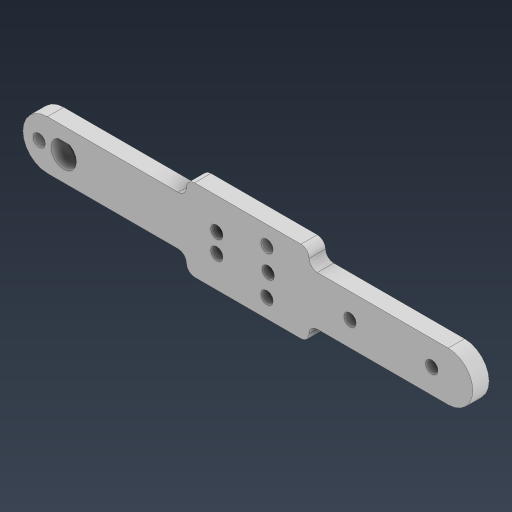
# Autodesk Inventor part: Arm1_3D
Saved by Autodesk Inventor 2023 (Build 270158000, 158)
## iProperties
Created: 2024-02-10
Part Number: Arm1_3D
Material: Generic
Document SubType Name: Modeling
Designer: victo
Density: 1 g/cm^3
Appearance: Default
Author: victo
Autodesk Inventor part; units mm, degrees
ref_plane "YZ Plane" through (0, 0, 0) normal (1, 0, 0) x (0, 1, 0)
ref_plane "XZ Plane" through (0, 0, 0) normal (0, 1, 0) x (-1, 0, 0)
ref_plane "XY Plane" through (0, 0, 0) normal (0, 0, 1) x (1, 0, 0)
sketch "Sketch1" plane through (0, 0, 0) normal (0, 0, 1) x (1, 0, 0)
  line L0 (0, 0) -> (90, 0) construction
  line L1 (0, -10) -> (90, -10)
  line L2 (90, 10) -> (0, 10)
  arc A0 (0, 10) -> (0, -10) centre (0, 0) ccw
  arc A1 (90, -10) -> (90, 10) centre (90, 0) ccw
  line L3 (0, 0) -> (90, 0) construction
  circle A2 centre (0, 0) radius 3.1
  circle A3 centre (-6, 0) radius 1.5
  circle A4 centre (0, 0) radius 37.5 construction
  circle A5 centre (0, 0) radius 50 construction
  circle A6 centre (37.4301, 2.2893) radius 1.5
  circle A7 centre (37.4301, -2.2893) radius 1.5
  circle A8 centre (50, 0) radius 1.5
  circle A9 centre (49.7028, 5.4433) radius 1.5
  circle A10 centre (49.7028, -5.4433) radius 1.5
  line L4 (37.4301, 2.2893) -> (0, 0) construction
  line L5 (0, 0) -> (49.7028, 5.4433) construction
  line L6 (37.4301, -2.2893) -> (0, 0) construction
  line L7 (49.7028, -5.4433) -> (0, 0) construction
  circle A11 centre (90, 0) radius 1.5
  line L8 (-10, 10) -> (10, 10)
  line L9 (10, 10) -> (10, -10)
  line L10 (10, -10) -> (-10, -10)
  line L11 (-10, -10) -> (-10, 10)
  line L12 (-10, 10) -> (10, -10) construction
  line L13 (10, 10) -> (-10, -10) construction
  line L14 (80, 10) -> (100, 10)
  line L15 (100, 10) -> (100, -10)
  line L16 (100, -10) -> (80, -10)
  line L17 (80, -10) -> (80, 10)
  line L18 (80, 10) -> (100, -10) construction
  line L19 (100, 10) -> (80, -10) construction
  line L20 (30, 10) -> (60, 10)
  line L21 (60, 10) -> (60, -10)
  line L22 (60, -10) -> (30, -10)
  line L23 (30, -10) -> (30, 10)
  line L24 (30, 10) -> (60, -10) construction
  line L25 (60, 10) -> (30, -10) construction
  line L26 (-10, 6) -> (100, 6)
  line L27 (100, 6) -> (100, -6)
  line L28 (100, -6) -> (-10, -6)
  line L29 (-10, -6) -> (-10, 6)
  line L30 (-10, 6) -> (100, -6) construction
  line L31 (100, 6) -> (-10, -6) construction
  line L32 (-1.478, 2.725) -> (1.478, 2.725)
  circle A12 centre (70, 0) radius 1.5
  point P0 (45, 0)
  point P1 (30, 6)
  point P2 (30, -6)
  point P3 (60, -6)
  point P4 (60, 6)
  dimension "d0" = 90
  dimension "d1" = 0
  dimension "d2" = 20
  dimension "d4" = 6.2
  dimension "d5" = 3
  dimension "d6" = 6
  dimension "d7" = 0
  dimension "d8" = 75
  dimension "d9" = 100
  dimension "d10" = 3
  dimension "d11" = 3
  dimension "d12" = 3
  dimension "d13" = 3
  dimension "d14" = 3
  dimension "d15" = 3.5
  dimension "d16" = 3.5
  dimension "d17" = 6.25
  dimension "d18" = 6.25
  dimension "d19" = 3
  dimension "d22" = 20
  dimension "d23" = 20
  dimension "d24" = 20
  dimension "d25" = 20
  dimension "d26" = 30
  dimension "d27" = 20
  dimension "d28" = 12
  dimension "d31" = 2.725
  dimension "d32" = 3
  dimension "d33" = 20
  dimension "d34" = 0
  constraints: 68 end point, 13 centre point, 11 point on circle, 9 midpoint, 9 parallel, 7 horizontal, 4 coincident, 4 perpendicular, 4 tangent, 2 point on line, 1 collinear
  measures "d0" distance of L0.start L0.end
  measures "d1" distance between parallel lines of L0 L3
  measures "d2" diameter of A1
  measures "d4" diameter of A2
  measures "d5" diameter of A3
  measures "d6" distance of L0.start A3.centre
  measures "d7" vertical distance of A3.centre L0.start
  measures "d8" diameter of A4
  measures "d9" diameter of A5
  measures "d10" diameter of A6
  measures "d11" diameter of A7
  measures "d12" diameter of A8
  measures "d13" diameter of A9
  measures "d14" diameter of A10
  measures "d15" angle of L0 L4
  measures "d16" angle of L0 L6
  measures "d17" angle of L3 L5
  measures "d18" angle of L0 L7
  measures "d19" diameter of A11
  measures "d22" distance of L9.end L10.end
  measures "d23" distance of L8.end L9.end
  measures "d24" distance of L15.end L16.end
  measures "d25" distance of L14.end L15.end
  measures "d26" distance of L21.end L22.end
  measures "d27" distance of L20.end L21.end
  measures "d28" distance of L26.end L27.end
  measures "d31" distance from line of A2.centre L32
  measures "d32" diameter of A12
  measures "d33" distance of A12.centre L0.end
  measures "d34" vertical distance of L0.end A12.centre
extrude "Extrusion1" add sketch "Sketch1" along normal blind 4 contours L28 L11 A0 | A0 L26 L9 L28 | L23 L28 A10 L21 L1 | L9 L26 L23 L28 | L11 L26 A0 | L23 L26 A9 L21 L28 A10 | L21 L26 L17 L28 | L23 L2 L21 L26 A9 | L17 L26 A1 L28 | A1 L15 L28 | A1 L26 L15 | L32 A2 picked at (0.2541, 2.8183)
fillet "Fillet1" radius 2 8 edges at (30, 6, 2) (30, 10, 2) (60, 10, 2) (60, 6, 2) (60, -6, 2) (60, -10, 2) (30, -10, 2) (30, -6, 2)
fillet "Fillet1" radius 6 4 edges at (-10, -6, 2) (-10, 6, 2) (100, -6, 2) (100, 6, 2)
sketch "Sketch2" plane through (0, 0, 4) normal (0, 0, 1) x (1, 0, 0)
  arc A0 (94, -6) -> (94, 6) centre (94, 0) ccw projected
  line L0 (94, 6) -> (62, 6) projected
  arc A1 (60, 8) -> (62, 6) centre (62, 8) ccw projected
  arc A2 (60, 8) -> (58, 10) centre (58, 8) ccw projected
  line L1 (58, 10) -> (32, 10) projected
  arc A3 (32, 10) -> (30, 8) centre (32, 8) ccw projected
  arc A4 (28, 6) -> (30, 8) centre (28, 8) ccw projected
  line L2 (28, 6) -> (-4, 6) projected
  arc A5 (-4, 6) -> (-4, -6) centre (-4, 0) ccw projected
  line L3 (-4, -6) -> (28, -6) projected
  arc A6 (30, -8) -> (28, -6) centre (28, -8) ccw projected
  arc A7 (30, -8) -> (32, -10) centre (32, -8) ccw projected
  line L4 (32, -10) -> (58, -10) projected
  arc A8 (58, -10) -> (60, -8) centre (58, -8) ccw projected
  arc A9 (62, -6) -> (60, -8) centre (62, -8) ccw projected
  line L5 (62, -6) -> (94, -6) projected
  circle A10 centre (90, 0) radius 1.5 projected
  circle A11 centre (70, 0) radius 1.5 projected
  circle A12 centre (49.7028, 5.4433) radius 1.5 projected
  circle A13 centre (50, 0) radius 1.5 projected
  circle A14 centre (37.4301, -2.2893) radius 1.5 projected
  circle A15 centre (37.4301, 2.2893) radius 1.5 projected
  circle A16 centre (-6, 0) radius 1.5 projected
  circle A17 centre (49.7028, -5.4433) radius 1.5 projected
  line L6 (-1.478, 2.725) -> (1.478, 2.725) projected
  arc A18 (-1.478, 2.725) -> (1.478, 2.725) centre (0, 0) ccw projected
body "Solid1"
